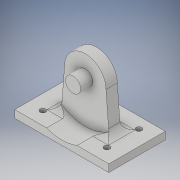
# Autodesk Inventor part: bearing support
Saved by Autodesk Inventor 2017 (Build 210142000, 142)
## iProperties
Created: 2017-04-10
Part Number: bearing support
Material: Generic
Document SubType Name: Modeling
Designer: Andres Celi
Density: 1 g/cm^3
Appearance: Default
Author: Andres Celi
Autodesk Inventor part; units mm, degrees
ref_plane "YZ Plane" through (0, 0, 0) normal (1, 0, 0) x (0, 1, 0)
ref_plane "XZ Plane" through (0, 0, 0) normal (0, 1, 0) x (-1, 0, 0)
ref_plane "XY Plane" through (0, 0, 0) normal (0, 0, 1) x (1, 0, 0)
sketch "Sketch1" plane through (0, 0, 0) normal (0, 0, 1) x (1, 0, 0)
  arc A0 (11, 0) -> (-11, 0) centre (0, 0) ccw
  line L0 (-11, 0) -> (11, 0)
  line L1 (0, 0) -> (0, -25)
  line L2 (-13, -25) -> (13, -25)
  line L3 (-11, 0) -> (-13, -25)
  line L4 (11, 0) -> (13, -25)
  dimension "d0" = 22
  dimension "d1" = 25
  dimension "d2" = 13
  dimension "d3" = 13
  constraints: 10 end point, 2 horizontal, 2 point on circle, 1 centre point, 1 coincident, 1 vertical
  measures "d0" diameter of A0
  measures "d1" distance of L1.start L1.end
  measures "d2" distance of L2.start L1.end
  measures "d3" distance of L1.end L2.end
extrude "Extrusion1" add sketch "Sketch1" along normal blind 6
sketch "Sketch2" plane through (0, 0, 6) normal (0, 0, 1) x (1, 0, 0)
  circle A0 centre (0, 0) radius 4
  dimension "d6" = 8
  constraints: 1 centre point, 1 coincident
  measures "d6" diameter of A0
extrude "Extrusion2" add sketch "Sketch2" along normal blind 6.5
sketch "Sketch3" plane through (-13, -25, 0) normal (0, -1, 0) x (1, 0, 0)
  line L0 (-12, 18.5) -> (38, 18.5)
  line L1 (38, 18.5) -> (38, -11.5)
  line L2 (38, -11.5) -> (-12, -11.5)
  line L3 (-12, -11.5) -> (-12, 18.5)
  point P0 (13, 0)
  dimension "d9" = 50
  dimension "d10" = 30
  dimension "d11" = 25
  dimension "d12" = 18.5
  constraints: 8 end point, 2 parallel, 1 horizontal, 1 perpendicular
  measures "d9" distance of L1.end L2.end
  measures "d10" distance of L0.end L1.end
  measures "d11" distance from line of L3 point (13, 0)
  measures "d12" distance from line of point (13, 0) L0
extrude "Extrusion3" add sketch "Sketch3" against normal blind 4
fillet "Fillet1" radius 4 4 edges at (0, -21, 6) (0, -21, 0) (-12.68, -21, 3) (12.68, -21, 3)
sketch "Sketch4" plane through (-25, -25, 18.5) normal (0, -1, 0) x (1, 0, 0)
  point P0 (25, -18.5)
sketch "Sketch5" plane through (-13, -21, 0) normal (0, 1, 0) x (1, 0, 0)
  circle A0 centre (30, 5.5) radius 1.5
  circle A1 centre (30, -11.5) radius 1.5
  circle A2 centre (-4, -11.5) radius 1.5
  circle A3 centre (-4, 5.5) radius 1.5
  line L0 (38, -18.5) -> (38, 11.5) projected
  line L1 (38, 11.5) -> (-12, 11.5) projected
  line L2 (-12, 11.5) -> (-12, -18.5) projected
  line L3 (-12, -18.5) -> (38, -18.5) projected
  point P0 (13, 0)
  dimension "d16" = 3
  dimension "d17" = 3
  dimension "d18" = 3
  dimension "d19" = 3
  dimension "d20" = 8
  dimension "d21" = 6
  dimension "d22" = 6
  dimension "d23" = 8
  dimension "d24" = 8
  dimension "d25" = 7
  dimension "d26" = 7
  dimension "d27" = 8
  constraints: 4 centre point
  measures "d16" diameter of A0
  measures "d17" diameter of A1
  measures "d18" diameter of A2
  measures "d19" diameter of A3
  measures "d20" distance from line of L0 A0.centre
  measures "d21" distance from line of L1 A0.centre
  measures "d22" distance from line of L1 A3.centre
  measures "d23" distance from line of L2 A3.centre
  measures "d24" distance from line of L2 A2.centre
  measures "d25" distance from line of L3 A2.centre
  measures "d26" distance from line of L3 A1.centre
  measures "d27" distance from line of L0 A1.centre
sketch "Sketch6" plane through (-13, -21, 0) normal (0, 1, 0) x (1, 0, 0)
  point P0 (13, 0)
extrude "Extrusion4" cut sketch "Sketch5" against normal blind 10 contours A0 | A1 | A2 | A3
sketch "Sketch7" plane through (0, 0, 12.5) normal (0, 0, 1) x (1, 0, 0)
  circle A0 centre (0, 0) radius 22.5
  circle A1 centre (0, 0) radius 4
  dimension "d30" = 45
  dimension "d31" = 8
  constraints: 2 centre point, 2 coincident
  measures "d30" diameter of A0
  measures "d31" diameter of A1
extrude "Extrusion5" cut sketch "Sketch7" along normal mid plane 13
body "Solid1"
